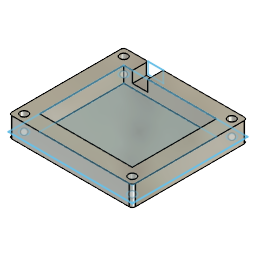
bottom (Autodesk Fusion 360 design; units mm, degrees)
part number: 2026-08-13-23-21-36-069
Autodesk Fusion 360 part; units mm, degrees
sketch "sketch 551" plane through (0, 0, 0) normal (0, 0, -1) x (1, 0, 0)
  line L0 (159.5512, 80) -> (80.0512, 80)
  line L1 (159.5512, 154) -> (159.5512, 80)
  line L2 (80.0512, 154) -> (159.5512, 154)
  line L3 (80.0512, 80) -> (80.0512, 154)
extrude "Extrude1" add sketch "sketch 551" along normal blind 3
sketch "sketch 573" plane through (0, 0, 0) normal (0, 0, -1) x (1, 0, 0)
  line L0 (149.5512, 90) -> (90.0512, 90)
  line L1 (90.0512, 90) -> (90.0512, 144)
  line L2 (90.0512, 144) -> (149.5512, 144)
  line L3 (149.5512, 144) -> (149.5512, 90)
  line L4 (159.5512, 80) -> (80.0512, 80)
  line L5 (159.5512, 154) -> (159.5512, 80)
  line L6 (80.0512, 154) -> (159.5512, 154)
  line L7 (80.0512, 80) -> (80.0512, 154)
extrude "Extrude2" add sketch "sketch 573" against normal blind 10
sketch "sketch 606" plane through (0, 0, 0) normal (0, 0, -1) x (1, 0, 0)
  circle A0 centre (154.5512, 85) radius 2.5
  circle A1 centre (85.0512, 149) radius 2.5
  circle A2 centre (154.5512, 149) radius 2.5
  circle A3 centre (85.0512, 85) radius 2.5
extrude "Extrude3" cut sketch "sketch 606" along normal blind 4 from surface at -10
sketch "sketch 630" plane through (0, -80, 0) normal (0, 1, 0) x (-1, 0, 0)
  line L0 (-95.685, 2.75) -> (-95.685, 10)
  line L1 (-95.685, 10) -> (-105.475, 10)
  line L2 (-95.685, 10) -> (-105.475, 10)
  line L3 (-105.475, 10) -> (-105.475, 2.75)
  line L4 (-105.475, 2.75) -> (-95.685, 2.75)
extrude "Extrude4" cut sketch "sketch 630" against normal blind 10
fillet "Fillet1" radius 2 4 edges at (159.5512, -154, 3.5) (159.5512, -80, 3.5) (80.0512, -154, 3.5) (80.0512, -80, 3.5)
fillet "Fillet2" radius 1 3 edges at (100.58, -80, 2.75) (95.685, -80, 6.375) (105.475, -80, 6.375)
